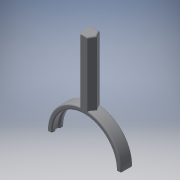
# Autodesk Inventor part: Magnifier Glass Holder Lower Half
Saved by Autodesk Inventor 2016 (Build 200138000, 138)
## iProperties
Created: 2014-08-03
Part Number: Magnifier Glass Holder Lower Half
Material: Generic
Document SubType Name: Modeling
Designer: steele
Density: 1 g/cm^3
Appearance: Default
Author: steele
Autodesk Inventor part; units mm, degrees
ref_plane "YZ Plane" through (0, 0, 0) normal (1, 0, 0) x (0, 1, 0)
sketch "Sketch1" plane through (0, 0, 0) normal (0, 0, 1) x (1, 0, 0)
  line L0 (0, 0) -> (50, 0) construction
  line L1 (50, 0) -> (50, 2)
  line L2 (55, 0) -> (55, 9)
  line L3 (55, 9) -> (48, 9)
  line L4 (48, 9) -> (48, 4)
  line L5 (48, 4) -> (50, 2)
  line L6 (50, 0) -> (55, 0) construction
  line L7 (50, 0) -> (50, -2)
  line L8 (55, 0) -> (55, -9)
  line L9 (55, -9) -> (48, -9)
  line L10 (48, -9) -> (48, -4)
  line L11 (48, -4) -> (50, -2)
  line L12 (0, -12.6) -> (0, 12.6) projected
  dimension "d0" = 50
  dimension "d1" = 9
  dimension "d2" = 5
  dimension "d3" = 7
  dimension "d4" = 5
  constraints: 24 end point, 4 symmetric about line, 3 perpendicular, 1 horizontal, 1 parallel
  measures "d0" distance of L0.start L0.end
  measures "d1" distance of L2.start L2.end
  measures "d2" distance between parallel lines of L1 L2
  measures "d3" distance of L2.end L3.end
  measures "d4" distance of L3.end L4.end
revolve "Revolution1" add sketch "Sketch1" angle 360 about axis through (0, -10, 0) along (0, 1, 0)
ref_plane "Work Plane1" through (0, 0, 50) normal (0, 0, 1) x (1, 0, 0)
sketch "Sketch2" plane through (0, 0, 50) normal (0, 0, 1) x (1, 0, 0)
  line L0 (5.1698, -9.0152) -> (-5.2225, -8.9847)
  line L1 (-5.2225, -8.9847) -> (-10.3923, 0.0304)
  line L2 (-10.3923, 0.0304) -> (-5.1698, 9.0152)
  line L3 (-5.1698, 9.0152) -> (5.2225, 8.9847)
  line L4 (5.2225, 8.9847) -> (10.3923, -0.0304)
  line L5 (10.3923, -0.0304) -> (5.1698, -9.0152)
  point P0 (0, 0)
  point P1 (0, 0)
  dimension "d23" = 18
  constraints: 12 end point, 13 other
  measures "d23" distance between parallel lines of L0 L3
extrude "Extrusion1" add sketch "Sketch2" along normal blind 100
fillet "Fillet2" radius 2 4 edges at (-37.0147, 9, -40.6806) (38.8955, 9, 38.8862) (-38.8862, -9, -38.8955) (40.6806, -9, 37.0147)
fillet "Fillet4" radius 2 2 edges at (-48, -9, 0) (-48, 9, 0)
fillet "Fillet5" radius 1 4 edges at (-48, -4, 0) (-50, -2, 0) (-48, 4, 0) (-50, 2, 0)
ref_plane "Work Plane2" through (0, 0, 0) normal (0, 0, 1) x (1, 0, 0)
sketch "Sketch3" plane through (0, 0, 0) normal (0, 1, 0) x (-1, 0, 0)
  line L0 (-60, 0) -> (60, 0)
  line L1 (60, 0) -> (60, -60)
  line L2 (60, -60) -> (-60, -60)
  line L3 (-60, -60) -> (-60, 0)
  point P0 (0, 0)
  constraints: 8 end point, 2 parallel, 1 horizontal, 1 perpendicular
extrude "Extrusion2" cut sketch "Sketch3" along normal mid plane 20
sketch "Sketch4" plane through (-50, -9, 0) normal (0, 0, -1) x (-1, 0, 0)
  line L0 (3, 0) -> (0, 0) projected
  line L1 (0, 18) -> (3, 18) projected
  line L2 (-2, 13.4142) -> (-2, 16) projected
  line L3 (-50, 27) -> (-50, -15) construction
  line L4 (1.5, 18) -> (1.5, 0) construction
  circle A0 centre (1.5, 14.5) radius 1.2402
  circle A1 centre (1.5, 3.5) radius 1.2402
  circle A2 centre (-101.5, 14.5) radius 1.2402
  circle A3 centre (-101.5, 3.5) radius 1.2402
  point P0 (-50, 9)
  dimension "d18" = 2.4805
  dimension "d19" = 3.5
  dimension "d20" = 3.5
  constraints: 4 centre point, 4 end point, 2 midpoint, 2 point on line, 2 symmetric about line, 1 equal radius, 1 parallel, 2 other
  measures "d18" diameter of A0
  measures "d19" distance from line of A0.centre L1
  measures "d20" distance from line of A1.centre L0
extrude "Extrusion3" cut sketch "Sketch4" against normal blind 6.985
fillet "Fillet8" radius 2 6 edges at (7.781, -4.5228, 150) (7.8074, 4.4771, 150) (0.0264, 9, 150) (-7.781, 4.5228, 150) (-7.8074, -4.4771, 150) (-0.0264, -9, 150)
body "Solid1"
